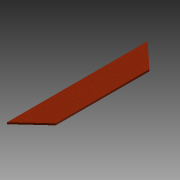
# Autodesk Inventor part: Ramp - End - Polycarbonated 125
Saved by Autodesk Inventor 2015 (Build 190159000, 159)
## iProperties
Created: 2015-01-21
Part Number: Ramp - End - Polycarbonated 125
Material: Wood (Oak)
Document SubType Name: Modeling
Designer: peters
Density: 0.76 g/cm^3
Appearance: White Oak - Natural Medium Gloss
Author: peters
Autodesk Inventor part; units mm, degrees
ref_plane "YZ Plane" through (0, 0, 0) normal (1, 0, 0) x (0, 1, 0)
ref_plane "XZ Plane" through (0, 0, 0) normal (0, 1, 0) x (-1, 0, 0)
ref_plane "XY Plane" through (0, 0, 0) normal (0, 0, 1) x (1, 0, 0)
sketch "Sketch1" plane through (0, 0, 0) normal (0, 1, 0) x (-1, 0, 0)
  line L0 (0, 0) -> (0, -508)
  line L1 (0, -508) -> (137.16, -635)
  line L2 (137.16, -635) -> (137.16, 127)
  line L3 (137.16, 127) -> (0, 0)
  dimension "d0" = 508
  dimension "d1" = 762
  dimension "d2" = 137.16
  constraints: 8 end point, 1 equal length, 1 parallel, 1 vertical
  measures "d0" distance of L0.start L0.end
  measures "d1" distance of L1.end L2.end
  measures "d2" distance between parallel lines of L0 L2
extrude "Extrusion1" add sketch "Sketch1" along normal blind 9.525
body "Solid1"
